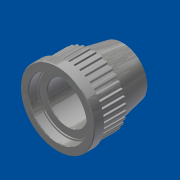
# Autodesk Inventor part: Synchronous Pulley1
Saved by Autodesk Inventor 2018 (Build 220112000, 112)
## iProperties
CustomPartVersion: 1
Created: 2019-11-13
Part Number: Synchronous Pulley1
Material: Steel
Document SubType Name: Modeling
Designer: Bunny320
Density: 1 g/cm^3
Appearance: Steel
Author: Bunny320
## iProperties of the stored document Synchronous Pulley1_3DPrint.ipt
Created: 2019-11-26
Part Number: Synchronous Pulley1_3DPrint
Material: Generic
Document SubType Name: Modeling
Designer: Bunny320
Density: 1 g/cm^3
Appearance: Default
Author: Bunny320
Autodesk Inventor part; units mm, degrees
ref_plane "YZ Plane" through (0, 0, 0) normal (1, 0, 0) x (0, 1, 0)
ref_plane "XZ Plane" through (0, 0, 0) normal (0, 1, 0) x (-1, 0, 0)
ref_plane "XY Plane" through (0, 0, 0) normal (0, 0, 1) x (1, 0, 0)
sketch "Pulley Sketch" plane through (0, 0, 0) normal (0, 0, 1) x (1, 0, 0)
  circle A0 centre (0, 0) radius 28.6479 construction
  circle A1 centre (0, 0) radius 28.1479
  circle A2 centre (0, 0) radius 26.8979
  line L0 (-1.4651, 28.1097) -> (-0.9, 26.8979)
  line L1 (-0.9, 26.8979) -> (0.9, 26.8979)
  line L2 (0.9, 26.8979) -> (1.4651, 28.1097)
  line L3 (0, 0) -> (0, 28.1479) construction
  point P0 (0, 26.8979)
  dimension "d0" = 57.2958
  dimension "d1" = 0.5
  dimension "d2" = 1.25
  dimension "d3" = 50
  dimension "d4" = 1.8
  constraints: 8 end point, 3 coincident, 3 point on circle, 2 centre point, 1 horizontal, 1 midpoint, 1 point on line, 1 vertical, 1 vertical alignment, 3 other
  measures "d0" diameter of A0
  measures "d1" radial gap between concentric circles of A0 A1
  measures "d3" angle of L2 L0
  measures "d4" distance of L0.end L1.end
extrude "Base Body" add sketch "Pulley Sketch" along normal mid plane 55 contours A2 | A1 L0 L1 L2 | L2 L1 L0 A1
extrude "Tooth" cut sketch "Pulley Sketch" along normal through all both and the other way through all contours L2 L1 L0 A1 picked at (0, 27.7284)
fillet "Tooth Fillet" radius 0.4 2 edges at (0.9, 26.8979, 0) (-0.9, 26.8979, 0)
fillet "Tooth Fillet" radius 0.6 4 edges at (-1.4651, 28.1097, 13.75) (-1.4651, 28.1097, -13.75) (1.4651, 28.1097, 13.75) (1.4651, 28.1097, -13.75)
pattern_circular "Teeth" count 36 over 360 about axis through (0, 0, -10) along (0, 0, 1) of "Tooth", "Tooth Fillet"
feature "Left flange" [suppressed]
feature "Right flange" [suppressed]
sketch "Sketch2" plane through (0, 0, 0) normal (0, 0, 1) x (1, 0, 0)
  point P0 (0, 0)
  point P1 (0, 0)
  constraints: 1 coincident
hole "Hole1" at (0, 0, 0) direction (0, 0, -1) diameter 6.5 end through all both
sketch "Sketch5" plane through (0, 0, -27.5) normal (0, 0, -1) x (-1, 0, 0)
  point P0 (0, 0)
  point P1 (9.9, 0)
  dimension "d34" = 9.9
  measures "d34" distance of point (0, 0) point (9.9, 0)
hole "Hole2" at (-9.9, 0, -27.5) direction (0, 0, 1) diameter 3.4 end through all countersink diameter 7.5 countersink angle 90 clearance for "Countersunk Flat Head Hex Socket Screw DIN EN ISO 10642" size "M3" standard "DIN"
pattern_circular "Circular Pattern2" count 6 over 360 about axis through (0, 0, 0) along (0, 0, 1) of "Hole2"
move faces "Move1" translate (0, 0, -2) faces at (0.2151, 15.6396, 27.5)
sketch "Sketch7" plane through (0, 0, 25.5) normal (0, 0, 1) x (1, 0, 0)
  circle A0 centre (0, 0) radius 23.55
  dimension "d52" = 47.1
  constraints: 1 centre point, 1 coincident
  measures "d52" diameter of A0
extrude "Extrusion5" cut sketch "Sketch7" against normal blind 7
sketch "Sketch8" plane through (0, 0, 18.5) normal (0, 0, 1) x (1, 0, 0)
  circle A0 centre (0, 0) radius 16.25
  dimension "d55" = 32.5
  constraints: 1 centre point, 1 coincident
  measures "d55" diameter of A0
extrude "Extrusion6" cut sketch "Sketch8" against normal blind 39
sketch "Sketch9" plane through (0, 0, -27.5) normal (0, 0, -1) x (-1, 0, 0)
  circle A0 centre (0, 0) radius 20
  circle A1 centre (0, 0) radius 38.6622
  dimension "d58" = 40
  constraints: 2 centre point, 2 coincident
  measures "d58" diameter of A0
extrude "Extrusion7" cut sketch "Sketch9" against normal blind 25
chamfer "Chamfer2" distance 25 distance2 5 1 edges at (20, 0, -2.5) measured on face at (20, 0, -3)
sketch "Sketch10" plane through (0, 0, 18.5) normal (0, 0, 1) x (1, 0, 0)
  circle A0 centre (0, 0) radius 22.5
  dimension "d64" = 45
  constraints: 1 centre point, 1 coincident
  measures "d64" diameter of A0
extrude "Extrusion8" cut sketch "Sketch10" against normal blind 1
sketch "Sketch12" plane through (0, 0, 25.5) normal (0, 0, 1) x (0.9961947, -0.0871557, 0)
  circle A0 centre (0, 0) radius 25
  circle A1 centre (0, 0) radius 30
  dimension "d70" = 60
  dimension "d71" = 50
  constraints: 2 centre point, 2 coincident
  measures "d70" diameter of A1
  measures "d71" diameter of A0
extrude "Extrusion9" add sketch "Sketch12" against normal blind 8
chamfer "Chamfer3" distance 0.5 angle 45 3 edges at (-23.55, 0, 25.5) (-16.25, 0, 17.5) (-29.8858, 2.6147, 25.5)
equation "\"d1\" = da_a"
equation "\"d2\" = da_hg"
equation "\"d3\" = 2 * da_fi"
equation "\"d4\" = da_bw"
equation "\"d5\" = da_bf"
equation "\"d7\" = da_bf"
equation "\"d9\" = da_rb"
equation "\"d10\" = da_rt"
equation "\"da_pb\" = 5"
equation "\"da_fi\" = 25deg"
equation "\"da_hg\" = 1.25"
equation "\"da_bw\" = 1.8"
equation "\"da_rb\" = 0.4"
equation "\"da_rt\" = 0.6"
equation "\"da_a\" = 0.5"
equation "\"da_bf\" = 55"
equation "\"da_wf\" = 1.5"
equation "\"da_hf\" = 1.5"
body "Solid1"
